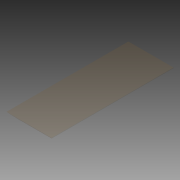
# Autodesk Inventor part: polycarb apendage bottom
Saved by Autodesk Inventor 2012 (Build 160160000, 160)
## iProperties
Created: 2013-07-07
Part Number: polycarb apendage bottom
Material: Default
Document SubType Name: Modeling
Designer: Bryce
Density: 1 g/cm^3
Author: Bryce
Autodesk Inventor part; units mm, degrees
ref_plane "YZ Plane" through (0, 0, 0) normal (1, 0, 0) x (0, 1, 0)
ref_plane "XZ Plane" through (0, 0, 0) normal (0, 1, 0) x (-1, 0, 0)
ref_plane "XY Plane" through (0, 0, 0) normal (0, 0, 1) x (1, 0, 0)
sketch "Sketch1" plane through (0, 0, 0) normal (0, 0, 1) x (1, 0, 0)
  line L0 (0, 0) -> (-196.1236, 0)
  line L1 (-254, 3.175) -> (0, 3.175)
  line L2 (0, 3.175) -> (0, 0)
  line L3 (-254, 3.175) -> (-196.1236, 0)
  dimension "d1" = 254
  dimension "d2" = 3.175
  dimension "d3" = 3.14
  constraints: 8 end point, 1 coincident, 1 horizontal, 1 parallel, 1 perpendicular
  measures "d1" distance of L1.start L1.end
  measures "d2" distance between parallel lines of L1 L0
  measures "d3" angle of L1 L3
extrude "Extrusion1" add sketch "Sketch1" along normal blind 685.8
body "Solid1"
